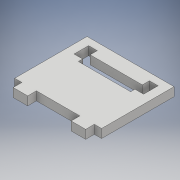
# Autodesk Inventor part: attache
Saved by Autodesk Inventor 2017 (Build 210142000, 142)
## iProperties
Part Number: attache
Material: Générique
Document SubType Name: Modeling
Designer: Thomas
Density: 1 g/cm^3
Appearance: Par défaut
Author: Thomas
Autodesk Inventor part; units mm, degrees
ref_plane "YZ Plane" through (0, 0, 0) normal (1, 0, 0) x (0, 1, 0)
ref_plane "XZ Plane" through (0, 0, 0) normal (0, 1, 0) x (-1, 0, 0)
ref_plane "XY Plane" through (0, 0, 0) normal (0, 0, 1) x (1, 0, 0)
sketch "Esquisse1" plane through (0, 0, 0) normal (0, 0, 1) x (1, 0, 0)
  line L0 (18.0239, 8.4751) -> (18.0239, 58.4751)
  line L1 (18.0239, 58.4751) -> (-41.9761, 58.4751)
  line L2 (-41.9761, 58.4751) -> (-41.9761, 8.4751)
  line L3 (-30.0261, 48.5751) -> (6.0739, 48.5751)
  line L4 (6.0739, 48.5751) -> (6.0739, 40.4751)
  line L5 (6.0739, 40.4751) -> (-30.0261, 40.4751)
  line L6 (-30.0261, 40.4751) -> (-30.0261, 48.5751)
  line L7 (-36.9761, 2.4751) -> (-36.9761, 8.4751)
  line L8 (-26.9761, 8.4751) -> (-26.9761, 2.4751)
  line L9 (3.0239, 8.4751) -> (3.0239, 2.4751)
  line L10 (13.0239, 8.4751) -> (13.0239, 2.4751)
  line L11 (-41.9761, 8.4751) -> (-36.9761, 8.4751)
  line L12 (13.0239, 8.4751) -> (18.0239, 8.4751)
  line L13 (-26.9761, 8.4751) -> (3.0239, 8.4751)
  line L14 (-36.9761, 2.4751) -> (-26.9761, 2.4751)
  line L15 (3.0239, 2.4751) -> (13.0239, 2.4751)
  line L16 (-35.9761, 53.4751) -> (-29.9761, 53.4751)
  line L17 (-29.9761, 53.4751) -> (-29.9761, 43.4751)
  line L18 (-29.9761, 43.4751) -> (-35.9761, 43.4751)
  line L19 (-35.9761, 43.4751) -> (-35.9761, 53.4751)
  line L20 (6.0239, 53.4751) -> (12.0239, 53.4751)
  line L21 (12.0239, 53.4751) -> (12.0239, 43.4751)
  line L22 (12.0239, 43.4751) -> (6.0239, 43.4751)
  line L23 (6.0239, 43.4751) -> (6.0239, 53.4751)
  point P0 (0, 0)
  dimension "d0" = 50
  dimension "d3" = 8.1
  dimension "d4" = 36.1
  dimension "d5" = 11.95
  dimension "d6" = 10
  dimension "d7" = 10
  dimension "d12" = 6
  dimension "d13" = 10
  dimension "d14" = 6
  dimension "d16" = 36
  dimension "d17" = 6
  dimension "d20" = 35
  dimension "d21" = 35
  dimension "d22" = 10
  dimension "d23" = 6
  dimension "d24" = 6
  dimension "d25" = 32
  constraints: 48 end point, 14 perpendicular, 10 parallel, 3 horizontal, 2 point on line
  measures "d0" distance of L0.end L0.start
  measures "d3" distance of L3.end L4.end
  measures "d4" distance of L3.start L3.end
  measures "d5" distance between parallel lines of L2 L6
  measures "d6" distance between parallel lines of L8 L7
  measures "d7" distance between parallel lines of L10 L9
  measures "d12" distance of L16.start L16.end
  measures "d13" distance of L16.end L17.end
  measures "d14" distance of L20.start L20.end
  measures "d16" distance between parallel lines of L23 L17
  measures "d17" distance between parallel lines of L19 L2
  measures "d20" distance between parallel lines of L11 L18
  measures "d21" distance between parallel lines of L12 L22
  measures "d22" distance between parallel lines of L22 L20
  measures "d23" distance of L7.start L7.end
  measures "d24" distance of L8.start L8.end
  measures "d25" distance between parallel lines of L13 L5
extrude "Extrusion1" add sketch "Esquisse1" along normal blind 6
